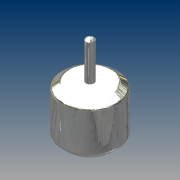
# Autodesk Inventor part: MotorTop
Saved by Autodesk Inventor 2011 SP1 (Build 150282100, 282)
## iProperties
Created: 2011-07-19
Part Number: MotorTop
Document SubType Name: Modeling
Designer: Nathan
Density: 1 g/cm^3
Author: Nathan
Autodesk Inventor part; units mm, degrees
ref_plane "YZ Plane" through (0, 0, 0) normal (1, 0, 0) x (0, 1, 0)
ref_plane "XZ Plane" through (0, 0, 0) normal (0, 1, 0) x (-1, 0, 0)
ref_plane "XY Plane" through (0, 0, 0) normal (0, 0, 1) x (1, 0, 0)
sketch "Sketch1" plane through (0, 0, 0) normal (0, 0, 1) x (1, 0, 0)
  line L0 (0, 43.18) -> (0, 0)
  line L1 (-10.3763, 25.4) -> (-2, 25.4)
  line L2 (-2, 25.4) -> (-2, 43.18)
  line L3 (-2, 43.18) -> (0, 43.18)
  line L4 (0, 0) -> (-10.3763, 0)
  line L5 (-10.3763, 0) -> (-13.97, 3.466)
  line L6 (-13.97, 3.466) -> (-13.97, 22.9252)
  line L7 (-13.97, 22.9252) -> (-10.3763, 25.4)
  point P0 (0, 21.59)
  dimension "d18" = 2
  dimension "d19" = 17.78
  dimension "d23" = 25.4
  dimension "d25" = 13.97
  constraints: 16 end point, 3 perpendicular, 2 parallel, 1 midpoint, 1 vertical, 1 other
  measures "d18" distance between parallel lines of L0 L2
  measures "d19" distance of L1.end L2.end
  measures "d23" distance between parallel lines of L4 L1
  measures "d25" distance between parallel lines of L0 L6
revolve "Revolution1" add sketch "Sketch1" angle 360 about axis through (0, 43.18, 0) along (0, -1, 0)
fillet "Fillet3" radius 1.5875 1 edges at (10.3763, 25.4, 0)
fillet "Fillet4" radius 1.5875 1 edges at (13.97, 22.9252, 0)
fillet "Fillet5" radius 1.5875 2 edges at (13.97, 3.466, 0) (10.3763, 0, 0)
body "Solid1"
